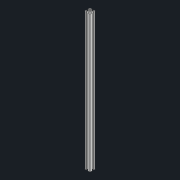
# Autodesk Inventor part: 8020
Saved by Autodesk Inventor 2022.3 (Build 263350000, 350)
## iProperties
Created: 2022-11-01
Part Number: 8020
Material: Generic
Document SubType Name: Modeling
Designer: JARRETT
Density: 1 g/cm^3
Appearance: Default
Author: JARRETT
Autodesk Inventor part; units mm, degrees
ref_plane "YZ Plane" through (0, 0, 0) normal (1, 0, 0) x (0, 1, 0)
ref_plane "XZ Plane" through (0, 0, 0) normal (0, 1, 0) x (-1, 0, 0)
ref_plane "XY Plane" through (0, 0, 0) normal (0, 0, 1) x (1, 0, 0)
sketch "Sketch1" plane through (0, 0, 0) normal (0, 1, 0) x (-1, 0, 0)
  circle A0 centre (0, 0) radius 2.15
  line L0 (-10, 10) -> (10, 10)
  line L1 (10, 10) -> (10, -10)
  line L2 (10, -10) -> (-10, -10)
  line L3 (-10, -10) -> (-10, 10)
  line L4 (-10, 10) -> (10, -10) construction
  line L5 (10, 10) -> (-10, -10) construction
  line L6 (10, -2.5) -> (8.5267, -2.5)
  line L7 (8.5267, -2.5) -> (8.5267, -4.8839)
  line L8 (7.0482, -5.4963) -> (3.6, -2.0481)
  line L9 (3.6, -2.0481) -> (3.6, 2.0481)
  line L10 (3.6, 2.0481) -> (7.0482, 5.4963)
  line L11 (8.5267, 4.8839) -> (8.5267, 2.5)
  line L12 (8.5267, 2.5) -> (10, 2.5)
  line L13 (0, 0) -> (10, 0) construction
  arc A1 (8.5267, 4.8839) -> (7.0482, 5.4963) centre (7.6606, 4.8839) ccw
  arc A2 (7.0482, -5.4963) -> (8.5267, -4.8839) centre (7.6606, -4.8839) ccw
  point P0 (8.5267, -6.9748)
  point P1 (8.5267, 6.9748)
  point P2 (3.6, 0)
  dimension "d0" = 4.3
  dimension "d1" = 20
  dimension "d2" = 20
  dimension "d3" = 5
  dimension "d4" = 6.4
  dimension "d14" = 11.5
  constraints: 28 end point, 9 point on line, 5 parallel, 4 midpoint, 4 point on circle, 4 tangent, 3 centre point, 3 perpendicular, 2 horizontal, 1 coincident, 1 collinear, 1 equal radius
  measures "d0" diameter of A0
  measures "d1" distance of L1.end L2.end
  measures "d2" distance of L0.end L1.end
  measures "d3" distance between parallel lines of L6 L12
  measures "d4" distance between parallel lines of L9 L1
extrude "Extrusion1" add sketch "Sketch1" along normal blind 500
extrude "Extrusion2" cut sketch "Sketch1" along normal blind 500 contours L1 L6 L7 A2 L8 L9 L10 A1 L11 L12
pattern_circular "Circular Pattern1" count 4 over 360 about axis through (0, -10, 0) along (0, 1, 0) of "Extrusion2"
fillet "Fillet1" radius 2 4 edges at (-10, 250, -10) (10, 250, -10) (10, 250, 10) (-10, 250, 10)
equation "\"d7\" = d5"
equation "\"d5\" = 500"
body "Solid1"
